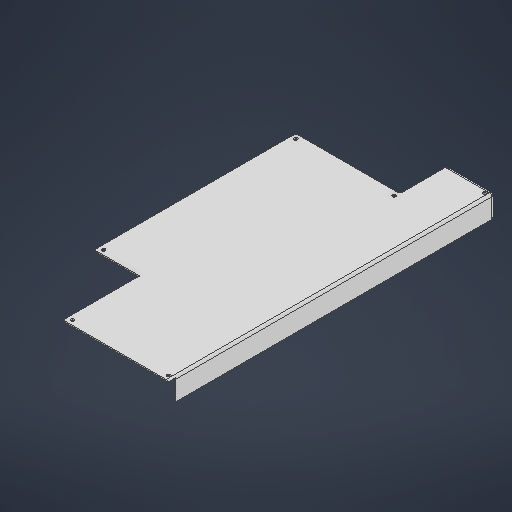
# Autodesk Inventor part: PCB_Qfab_Deckel
Saved by Autodesk Inventor 2027 (Build 310192060, 192F)
## iProperties
Created: 2026-06-09
Part Number: PCB_Qfab_Deckel
Material: Generisch
Document SubType Name: Modeling
Designer: simon
Density: 1 g/cm^3
Appearance: Vorgabe
Author: simon
Autodesk Inventor part; units mm, degrees
ref_plane "YZ Plane" through (0, 0, 0) normal (1, 0, 0) x (0, 1, 0)
ref_plane "XZ Plane" through (0, 0, 0) normal (0, 1, 0) x (-1, 0, 0)
ref_plane "XY Plane" through (0, 0, 0) normal (0, 0, 1) x (1, 0, 0)
sketch "Skizze2" plane through (0, 0, 0) normal (0, 0, 1) x (1, 0, 0)
  line L0 (91, -66) -> (91, 215.3)
  line L1 (91, -66) -> (0, -66)
  line L2 (0, -66) -> (0, 0)
  line L3 (91, 215.3) -> (51, 215.3)
  line L4 (51, 215.3) -> (51, 174)
  line L5 (51, 174) -> (-39, 174)
  line L6 (-39, 174) -> (-39, 0)
  line L7 (-39, 0) -> (0, 0)
  line L8 (0, 0) -> (91, 0) construction
  dimension "d0" = 281.3
  dimension "d1" = 91
  dimension "d2" = 66
  dimension "d3" = 40
  dimension "d4" = 41.3
  dimension "d5" = 90
  constraints: 18 end point, 4 perpendicular, 4 point on line, 2 horizontal, 2 vertical
  measures "d0" distance of L0.start L0.end
  measures "d1" distance of L0.start L1.end
  measures "d2" distance of L1.end L2.end
  measures "d3" distance of L0.end L3.end
  measures "d4" distance of L3.end L4.end
  measures "d5" distance of L4.end L5.end
extrude "Extrusion1" add sketch "Skizze2" along normal blind 1
sketch "Skizze3" plane through (0, 0, 1) normal (0, 0, 1) x (1, 0, 0)
  circle A0 centre (4, -62) radius 1.5
  line L0 (0, -66) -> (91, -66) projected
  line L1 (0, 0) -> (0, -66) projected
  circle A1 centre (87.122, -62) radius 1.5
  line L2 (91, -66) -> (91, 215.3) projected
  circle A2 centre (-35, 4) radius 1.5
  line L3 (-39, 0) -> (0, 0) projected
  line L4 (-39, 174) -> (-39, 0) projected
  circle A3 centre (-35, 170) radius 1.5
  line L5 (51, 174) -> (-39, 174) projected
  dimension "d8" = 3
  dimension "d9" = 4
  dimension "d10" = 4
  dimension "d11" = 4
  dimension "d12" = 3
  dimension "d13" = 3.878
  dimension "d14" = 3
  dimension "d15" = 4
  dimension "d16" = 4
  dimension "d17" = 3
  dimension "d18" = 4
  dimension "d19" = 4
  constraints: 4 centre point
  measures "d8" diameter of A0
  measures "d9" distance from line of L0 A0.centre
  measures "d10" distance from line of L1 A0.centre
  measures "d11" distance from line of L0 A1.centre
  measures "d12" diameter of A1
  measures "d13" distance from line of L2 A1.centre
  measures "d14" diameter of A2
  measures "d15" distance from line of L3 A2.centre
  measures "d16" distance from line of L4 A2.centre
  measures "d17" diameter of A3
  measures "d18" distance from line of L4 A3.centre
  measures "d19" distance from line of L5 A3.centre
extrude "Extrusion2" cut sketch "Skizze3" against normal blind 1.5
sketch "Skizze5" plane through (0, 0, 0) normal (0, 0, -1) x (-1, 0, 0)
  line L0 (0, -66) -> (-91, -66) projected
  line L1 (-91, 215.3) -> (-51, 215.3) projected
  line L2 (-91, -66) -> (-89.5, -66)
  line L3 (-89.5, -66) -> (-89.5, 215.3)
  line L4 (-89.5, 215.3) -> (-91, 215.3)
  line L5 (-91, 215.3) -> (-91, -66)
  line L6 (-51, 215.3) -> (-51, 174) projected
  line L7 (-91, 215.3) -> (-51, 215.3)
  line L8 (-51, 215.3) -> (-51, 213.8)
  line L9 (-51, 213.8) -> (-91, 213.8)
  line L10 (-91, 213.8) -> (-91, 215.3)
  point P0 (0, 0)
  point P1 (-89.5, 213.8)
  dimension "d36" = 1.5
  dimension "d43" = 1.5
  constraints: 16 end point, 4 parallel, 2 horizontal, 2 perpendicular, 2 point on line
  measures "d36" distance of L4.end L3.end
  measures "d43" distance of L7.end L8.end
extrude "Extrusion4" add sketch "Skizze5" along normal blind 17.9
sketch "Skizze6" plane through (91, -66, 1) normal (1, 0, 0) x (0, 0, -1)
  line L0 (0, 0) -> (18.9, 0) projected
  line L1 (18.9, 0) -> (18.9, 279.8) projected
  line L2 (1, 0) -> (18.9, 0)
  line L3 (18.9, 0) -> (18.9, 6.5)
  line L4 (18.9, 6.5) -> (1, 6.5)
  line L5 (1, 6.5) -> (1, 0)
  line L6 (1, 279.8) -> (1, 0) projected
  line L7 (18.9, 0) -> (18.9, 279.8) projected
  line L8 (1, 0) -> (18.9, 0) projected
  line L9 (1, 279.8) -> (18.9, 279.8) projected
  point P0 (1, 66)
  point P1 (18.4, 281.3)
  dimension "d39" = 6.5
  constraints: 8 end point, 2 parallel, 2 point on line, 1 horizontal, 1 perpendicular, 2 other
  measures "d39" distance of L4.end L2.start
extrude "Extrusion5" cut sketch "Skizze6" against normal blind 1.5 contours L5 L4 L1 L0
fillet "Rundung1" radius 2 7 edges at (91, 74.65, 1) (91, 215.3, -8.45) (71, 215.3, 1) (51, 174, 0.5) (-39, 174, 0.5) (-39, 0, 0.5) (0, -66, 0.5)
sketch "Skizze7" plane through (0, 0, 1) normal (0, 0, 1) x (1, 0, 0)
  line L0 (89, 215.3) -> (51, 215.3) projected
  line L1 (91, -59.5) -> (91, 213.3) projected
  line L2 (49, 174) -> (-37, 174) projected
  line L3 (51, 213.3) -> (51, 176) projected
  point P0 (0, 0)
  point P1 (87, 211.3)
  point P2 (50, 170)
  dimension "d44" = 4
  dimension "d45" = 4
  dimension "d53" = 4
  dimension "d54" = 1
  measures "d44" distance from line of L0 point (87, 211.3)
  measures "d45" distance from line of L1 point (87, 211.3)
  measures "d53" distance from line of L2 point (50, 170)
  measures "d54" distance from line of point (50, 170) L3
hole "Bohrung1" at (87, 211.3, 1) at (50, 170, 1) direction (0, 0, -1) diameter 3 depth 1
sketch "Skizze10" plane through (51, 215.3, -1) normal (0, 1, 0) x (1, 0, 0)
  line L0 (0, -1) -> (0, 16.9) projected
  line L1 (38.5, 16.9) -> (0, 16.9) projected
  line L2 (0, -1) -> (1.5, -1)
  line L3 (1.5, -1) -> (1.5, 16.9)
  line L4 (1.5, 16.9) -> (0, 16.9)
  line L5 (0, 16.9) -> (0, -1)
  point P0 (-51, -1)
  dimension "d58" = 1.5
  constraints: 8 end point, 2 parallel, 1 horizontal, 1 perpendicular, 1 point on line
  measures "d58" distance of L4.end L3.end
extrude "Extrusion7" cut sketch "Skizze10" against normal up to surface (1.5 mm away)
